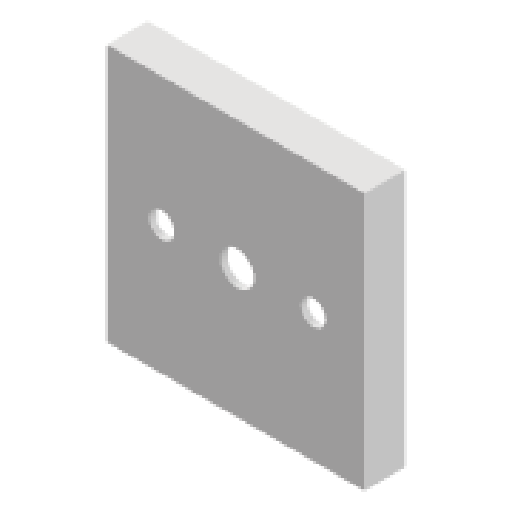
# Autodesk Inventor part: sensor_estructura
Saved by Autodesk Inventor 2025 (Build 290162000, 162)
## iProperties
Created: 2026-02-02
Part Number: sensor_estructura
Material: Genérico
Document SubType Name: Modeling
Designer: HP
Density: 1 g/cm^3
Appearance: Valor por defecto
Author: HP
Autodesk Inventor part; units mm, degrees
ref_plane "YZ Plane" through (0, 0, 0) normal (1, 0, 0) x (0, 1, 0)
ref_plane "XZ Plane" through (0, 0, 0) normal (0, 1, 0) x (-1, 0, 0)
ref_plane "XY Plane" through (0, 0, 0) normal (0, 0, 1) x (1, 0, 0)
sketch "Boceto4" plane through (0, 0, 0) normal (0, 0, 1) x (1, 0, 0)
  circle A0 centre (-1.0562, 12.2493) radius 5 projected
  line L0 (33.4438, -22.7507) -> (-36.5562, -22.7507) projected
  line L1 (33.4438, 47.2493) -> (33.4438, -22.7507) projected
  line L2 (-36.5562, 47.2493) -> (33.4438, 47.2493) projected
  line L3 (-36.5562, -22.7507) -> (-36.5562, 47.2493) projected
  circle A1 centre (21.3438, 12.2493) radius 3.7 projected
  circle A2 centre (-23.4562, 12.2493) radius 3.7 projected
  line L4 (36.4438, 50.2493) -> (-39.5562, 50.2493) projected
  line L5 (-39.5562, 50.2493) -> (-39.5562, -25.7507) projected
  line L6 (-39.5562, -25.7507) -> (36.4438, -25.7507) projected
  line L7 (36.4438, -25.7507) -> (36.4438, 50.2493) projected
  line L8 (33.4438, -22.7507) -> (-36.5562, -22.7507) projected
  line L9 (-36.5562, -22.7507) -> (-36.5562, 47.2493) projected
  line L10 (-36.5562, 47.2493) -> (33.4438, 47.2493) projected
  line L11 (33.4438, 47.2493) -> (33.4438, -22.7507) projected
  point P0 (0, 0)
extrude "Extrusión4" add sketch "Boceto4" against normal blind 10 contours L7 L6 L5 L4
sketch "Boceto5" plane through (0, 0, 0) normal (0, 0, 1) x (1, 0, 0)
  line L0 (-39.5562, 50.2493) -> (-39.5562, -25.7507) projected
  line L1 (-39.5562, -25.7507) -> (36.4438, -25.7507) projected
  line L2 (36.4438, -25.7507) -> (36.4438, 50.2493) projected
  line L3 (36.4438, 50.2493) -> (-39.5562, 50.2493) projected
  line L4 (-36.5562, -22.7507) -> (-36.5562, 47.2493) projected
  line L5 (-36.5562, 47.2493) -> (33.4438, 47.2493) projected
  line L6 (33.4438, 47.2493) -> (33.4438, -22.7507) projected
  line L7 (33.4438, -22.7507) -> (-36.5562, -22.7507) projected
  circle A0 centre (-1.0562, 12.2493) radius 5 projected
  line L8 (33.4438, -22.7507) -> (-36.5562, -22.7507) projected
  line L9 (33.4438, 47.2493) -> (33.4438, -22.7507) projected
  line L10 (-36.5562, 47.2493) -> (33.4438, 47.2493) projected
  line L11 (-36.5562, -22.7507) -> (-36.5562, 47.2493) projected
  circle A1 centre (21.3438, 12.2493) radius 3.7 projected
  circle A2 centre (-23.4562, 12.2493) radius 3.7 projected
  point P0 (0, 0)
extrude "Extrusión5" add sketch "Boceto5" along normal blind 2 contours L3 L2 L1 L0 | L4 L5 L6 L7
sketch "Boceto6" plane through (0, 0, 0) normal (0, 0, -1) x (-1, 0, 0)
  line L0 (39.5562, 50.2493) -> (-36.4438, 50.2493) projected
  line L1 (-36.4438, 50.2493) -> (-36.4438, -25.7507) projected
  line L2 (-36.4438, -25.7507) -> (39.5562, -25.7507) projected
  line L3 (39.5562, -25.7507) -> (39.5562, 50.2493) projected
  circle A0 centre (1.0562, 12.2493) radius 5 projected
  circle A1 centre (-21.3438, 12.2493) radius 3.7 projected
  circle A2 centre (23.4562, 12.2493) radius 3.7 projected
  circle A3 centre (5.2662, -1.7699) radius 1.5 projected
  circle A4 centre (-7.7338, -1.7699) radius 1.5 projected
  point P0 (0, 0)
extrude "Extrusión6" add sketch "Boceto6" against normal blind 2 contours A0 | A1 | A2
sketch "Boceto8" plane through (0, 0, 0) normal (0, 0, -1) x (-1, 0, 0)
  circle A0 centre (5.2662, -1.7699) radius 1.5 projected
  circle A1 centre (-7.7338, -1.7699) radius 1.5 projected
  point P0 (0, 0)
extrude "Extrusión7" cut sketch "Boceto8" against normal blind 2
